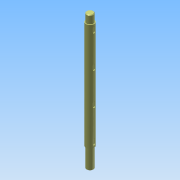
# Autodesk Inventor part: 装填盘轴
Saved by Autodesk Inventor 2015 (Build 190159000, 159)
## iProperties
Created: 2017-05-04
Part Number: 装填盘轴
Material: 常规
Document SubType Name: Modeling
Designer: Administrator
Density: 1 g/cm^3
Appearance: 缎光 - 柠檬绸色
Author: Administrator
Autodesk Inventor part; units mm, degrees
ref_plane "XZ Plane" through (0, 0, 0) normal (0, 1, 0) x (-1, 0, 0)
ref_plane "XY Plane" through (0, 0, 0) normal (0, 0, 1) x (1, 0, 0)
sketch "草图1" plane through (0, 0, 0) normal (0, 0, 1) x (1, 0, 0)
  circle A0 centre (0, 0) radius 15
  dimension "d0" = 30
  constraints: 1 centre point, 1 coincident
  measures "d0" diameter of A0
extrude "拉伸1" add sketch "草图1" against normal blind 398
ref_plane "工作平面1" through (15, 0, 0) normal (1, 0, 0) x (0, 1, 0)
sketch "草图2" plane through (15, 0, 0) normal (1, 0, 0) x (0, 1, 0)
  line L0 (4, -12) -> (-4, -12)
  line L1 (-4, -12) -> (-4, -26)
  line L2 (-4, -26) -> (4, -26)
  line L3 (4, -26) -> (4, -12)
  arc A0 (-4, -26) -> (4, -26) centre (0, -26) ccw
  arc A1 (4, -12) -> (-4, -12) centre (0, -12) ccw
  point P0 (0, 0)
  dimension "d3" = 8
  dimension "d4" = 14
  dimension "d5" = 0
  dimension "d6" = 12
  constraints: 8 end point, 4 point on circle, 4 tangent, 2 centre point, 2 parallel, 1 horizontal, 1 perpendicular
  measures "d3" distance of L1.end L2.end
  measures "d4" distance of L2.end L0.start
  measures "d5" horizontal distance of point (0, 0) A1.centre
  measures "d6" distance of point (0, 0) A1.centre
extrude "拉伸2" cut sketch "草图2" against normal blind 3
pattern_linear "矩形阵列1" count 4 spacing 120 along (0, 0, -1) of "拉伸2"
fillet "圆角1" radius 0.5 16 edges at (12, 0, -30) (12, -4, -19) (12, 0, -8) (12, 4, -19) (12, -4, -139) (12, 0, -128) (12, 4, -139) (12, 0, -150) (12, -4, -259) (12, 0, -248) (12, 4, -259) (12, 0, -270) (12, -4, -379) (12, 0, -368) (12, 4, -379) (12, 0, -390)
sketch "草图3" plane through (0, 0, -398) normal (0, 0, -1) x (-1, 0, 0)
  circle A0 centre (0, 0) radius 12.5
  dimension "d13" = 25
  constraints: 1 centre point, 1 coincident
  measures "d13" diameter of A0
extrude "拉伸3" add sketch "草图3" along normal blind 71
sketch "草图4" plane through (0, 0, 0) normal (0, 0, 1) x (1, 0, 0)
  circle A0 centre (0, 0) radius 12.5
  dimension "d16" = 25
  constraints: 1 centre point, 1 coincident
  measures "d16" diameter of A0
extrude "拉伸4" add sketch "草图4" along normal blind 30
chamfer "倒角1" distance 2 angle 45 1 edges at (-12.5, 0, 30)
